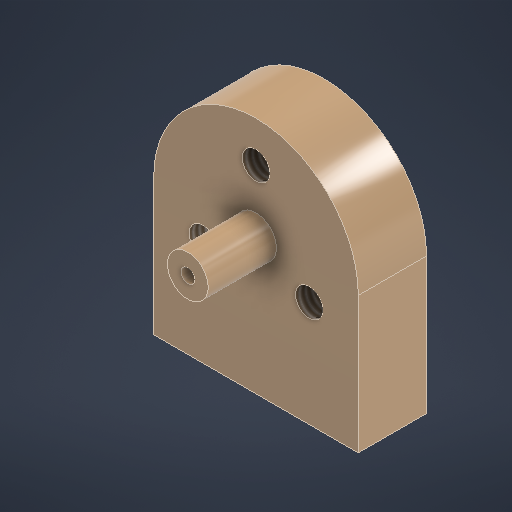
# Autodesk Inventor part: FillLine-SealFlange
Saved by Autodesk Inventor 2026 (Build 300175050, 175E)
## iProperties
Created: 2020-12-09
Part Number: FillLine-SealFlange
Material: Brass, Soft Yellow
Document SubType Name: Modeling
Designer: schanen
Density: 8.47 g/cm^3
Appearance: Brindle
Author: schanen
Autodesk Inventor part; units mm, degrees
ref_plane "YZ Plane" through (0, 0, 0) normal (1, 0, 0) x (0, 1, 0)
ref_plane "XZ Plane" through (0, 0, 0) normal (0, 1, 0) x (-1, 0, 0)
sketch "Sketch1" plane through (0, 0, 0) normal (0, 0, 1) x (1, 0, 0)
  line L0 (0, 0) -> (-15, 0)
  line L1 (-15, 0) -> (-15, 10)
  line L2 (-15, 10) -> (0, 10)
  line L3 (0, 10) -> (0, 0)
  circle A0 centre (-7.5, 10) radius 7.5
  dimension "d0" = 15
  dimension "d1" = 10
  constraints: 8 end point, 2 parallel, 1 horizontal, 1 midpoint, 1 perpendicular, 3 other
  measures "d0" distance of L1.end L2.end
  measures "d1" distance of L0.end L1.end
extrude "Extrusion1" add sketch "Sketch1" along normal blind 5
sketch "Sketch2" plane through (0, 0, 5) normal (0, 0, 1) x (1, 0, 0)
  arc A0 (0, 10) -> (-15, 10) centre (-7.5, 10) ccw projected
  circle A1 centre (-7.5, 10) radius 1.5
  point P0 (0, 0)
  dimension "d4" = 3
  constraints: 1 centre point, 1 coincident
  measures "d4" diameter of A1
extrude "Extrusion2" add sketch "Sketch2" along normal blind 5
sketch "Sketch3" plane through (-7.5, 10, 10) normal (0, 0, 1) x (1, 0, 0)
  point P0 (7.5, -10)
  point P1 (0, 0)
  point P2 (0, 0)
  constraints: 1 coincident
hole "Hole1" at (-7.5, 10, 10) direction (0, 0, -1) diameter 1 end through all
sketch "Sketch4" plane through (0, 0, 0) normal (0, 0, -1) x (-1, 0, 0)
  circle A0 centre (7.5, 10) radius 0.5 projected
  circle A1 centre (7.5, 10) radius 0.9
  point P0 (0, 0)
  dimension "d14" = 1.8
  constraints: 1 centre point, 1 coincident
  measures "d14" diameter of A1
extrude "Extrusion3" cut sketch "Sketch4" against normal blind 7 contours A0 | A1
sketch "Sketch5" plane through (0, 0, 0) normal (0, 0, -1) x (-1, 0, 0)
  circle A0 centre (7.5, 10) radius 0.9 projected
  circle A1 centre (7.5, 10) radius 1.5
  point P0 (0, 0)
  dimension "d17" = 3
  constraints: 1 centre point, 1 coincident
  measures "d17" diameter of A1
extrude "Extrusion4" cut sketch "Sketch5" against normal blind 1.5
sketch "Sketch7" plane through (-15, 0, 0) normal (0, -1, 0) x (1, 0, 0)
  line L0 (15, 0) -> (15, 5) projected
  line L1 (0, 0) -> (0, 5) projected
  line L2 (0, 0) -> (15, 0) projected
  point P0 (12, 2.5)
  point P1 (3, 2.5)
  dimension "d21" = 3
  dimension "d22" = 3
  dimension "d23" = 2.5
  dimension "d24" = 2.5
  measures "d21" distance from line of L0 point (12, 2.5)
  measures "d22" distance from line of L1 point (3, 2.5)
  measures "d23" distance from line of L2 point (12, 2.5)
  measures "d24" distance from line of L2 point (3, 2.5)
hole "Hole2" at (-3, 0, 2.5) at (-12, 0, 2.5) direction (0, 1, 0) diameter 2.013 depth 4 tip angle 118 thread size "M2.5x0.45" class "6H" standard "ISO Metric profile"
sketch "Sketch8" plane through (0, 0, 0) normal (0, 0, -1) x (-1, 0, 0)
  circle A0 centre (7.5, 10) radius 0.5 projected
  circle A1 centre (7.5, 10) radius 4.5 construction
  point P0 (0, 0)
  point P1 (7.5, 14.5)
  point P2 (11.3971, 7.75)
  point P3 (3.6029, 7.75)
  dimension "d32" = 9
  dimension "d33" = 120
  dimension "d34" = 120
  constraints: 3 point on circle, 1 centre point, 1 coincident
  measures "d32" diameter of A1
hole "Hole3" at (-7.5, 14.5, 0) at (-11.3971, 7.75, 0) at (-3.6029, 7.75, 0) direction (0, 0, 1) diameter 2.013 end through all thread size "M2.5x0.45" class "6H" standard "ISO Metric profile"
sketch "Sketch9" plane through (-7.5, 10, 10) normal (0, 0, 1) x (1, 0, 0)
  circle A0 centre (0, 0) radius 0.9 projected
  point P0 (7.5, -10)
  constraints: 1 coincident
ref_plane "Work Plane1" through (-7.5, 10, 10) normal (1, 0, 0) x (0, 0, -1)
body "Solid1"
